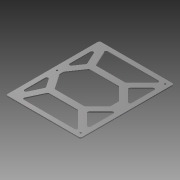
# Autodesk Inventor part: ZBedPlate
Saved by Autodesk Inventor 2015 SP1 (Build 190203100, 203)
## iProperties
Category: Sheet Metal
Created: 2015-01-11
Part Number: ZBedPlate
Material: Steel, Alloy
Document SubType Name: Modeling
Designer: Jack
Density: 7.73 g/cm^3
Appearance: Semi-Polished
Mass: 734.813 g
Surface Area: 727.52 cm^2
Volume: 95.0599 cm^3
Catalog Web Link: N/A
Author: Jack
Title: Bed Support Plate
Autodesk Inventor part; units mm, degrees
ref_plane "YZ Plane" through (0, 0, 0) normal (1, 0, 0) x (0, 1, 0)
ref_plane "XZ Plane" through (0, 0, 0) normal (0, 1, 0) x (-1, 0, 0)
ref_plane "XY Plane" through (0, 0, 0) normal (0, 0, 1) x (1, 0, 0)
sketch "Sketch1" plane through (0, 0, 0) normal (0, 0, 1) x (1, 0, 0)
  line L0 (0, 0) -> (236.5, 0)
  line L1 (236.5, 0) -> (236.5, 296)
  line L2 (236.5, 296) -> (0, 296)
  line L3 (0, 296) -> (0, 0)
  dimension "d0" = 236.5
  dimension "d1" = 296
  constraints: 8 end point, 2 parallel, 1 horizontal, 1 perpendicular
  measures "d0" distance of L0.start L0.end
  measures "d1" distance of L2.end L0.start
extrude "Extrusion1" add sketch "Sketch1" along normal blind 3
sketch "Sketch2" plane through (0, 0, 3) normal (0, 0, 1) x (1, 0, 0)
  line L0 (0, 0) -> (236.5, 0) projected
  line L1 (236.5, 0) -> (236.5, 296) projected
  line L2 (236.5, 296) -> (0, 296) projected
  line L3 (0, 296) -> (0, 0) projected
  line L4 (213.7907, 281) -> (33.7907, 281)
  line L5 (33.7907, 281) -> (60.8366, 223)
  line L6 (60.8366, 223) -> (155.5133, 223)
  line L7 (155.5133, 223) -> (213.7907, 281)
  line L8 (221.5, 260.4555) -> (173.8075, 212.9901)
  line L9 (173.8075, 212.9901) -> (221.5, 165.2976)
  line L10 (196.6646, 161.8487) -> (155.5133, 203)
  line L11 (221.5, 260.4555) -> (221.5, 165.2976)
  line L12 (155.5133, 203) -> (60.8366, 203)
  line L13 (60.8366, 203) -> (27.9297, 155)
  line L14 (15, 273.9728) -> (43.4367, 212.9901)
  line L15 (43.4367, 212.9901) -> (15, 171.5105)
  line L16 (15, 171.5105) -> (15, 273.9728)
  line L17 (27.9297, 141) -> (60.8366, 93)
  line L18 (60.8366, 93) -> (155.5133, 93)
  line L19 (155.5133, 93) -> (196.6646, 134.1513)
  line L20 (196.6646, 134.1513) -> (196.6646, 161.8487)
  line L21 (221.5, 130.7024) -> (173.8075, 83.0099)
  line L22 (173.8075, 83.0099) -> (221.5, 35.5445)
  line L23 (221.5, 35.5445) -> (221.5, 130.7024)
  line L24 (15, 124.4895) -> (43.4367, 83.0099)
  line L25 (43.4367, 83.0099) -> (15, 22.0272)
  line L26 (15, 22.0272) -> (15, 124.4895)
  line L27 (33.7907, 15) -> (213.7907, 15)
  line L28 (213.7907, 15) -> (155.5133, 73)
  line L29 (155.5133, 73) -> (60.8366, 73)
  line L30 (60.8366, 73) -> (33.7907, 15)
  line L31 (27.9297, 141) -> (27.9297, 155)
  dimension "d19" = 65
  dimension "d29" = 110
  dimension "d31" = 20
  dimension "d32" = 15
  dimension "d33" = 15
  dimension "d34" = 15
  dimension "d35" = 15
  dimension "d40" = 20
  dimension "d41" = 20
  dimension "d52" = 180
  dimension "d53" = 14
  dimension "d55" = 135
  dimension "d59" = 20
  dimension "d60" = 20
  dimension "d61" = 20
  dimension "d62" = 20
  dimension "d63" = 20
  constraints: 56 end point, 11 parallel, 9 vertical alignment, 8 equal length, 5 vertical, 4 horizontal, 2 horizontal alignment
  measures "d19" angle of L27 L30
  measures "d29" distance between parallel lines of L18 L12
  measures "d31" distance between parallel lines of L6 L12
  measures "d32" distance between parallel lines of L2 L4
  measures "d33" distance between parallel lines of L0 L27
  measures "d34" distance between parallel lines of L1 L11
  measures "d35" distance between parallel lines of L3 L16
  measures "d40" distance between parallel lines of L13 L15
  measures "d41" distance between parallel lines of L9 L10
  measures "d52" distance of L27.start L27.end
  measures "d53" distance of L17.start L13.end
  measures "d55" angle of L12 L10
  measures "d59" distance between parallel lines of L29 L18
  measures "d60" distance between parallel lines of L30 L25
  measures "d61" distance between parallel lines of L22 L28
  measures "d62" distance between parallel lines of L8 L7
  measures "d63" distance between parallel lines of L14 L5
extrude "Extrusion2" cut sketch "Sketch2" against normal up to next contours L7 L6 L5 L4 | L11 L9 L8 | L20 L19 L18 L17 L31 L13 L12 L10 | L14 L15 L16 | L23 L22 L21 | L24 L25 L26 | L30 L29 L28 L27
sketch "Sketch3" plane through (0, 0, 3) normal (0, 0, 1) x (1, 0, 0)
  line L0 (0, 0) -> (236.5, 0) projected
  line L1 (236.5, 0) -> (236.5, 296) projected
  line L2 (236.5, 296) -> (0, 296) projected
  line L3 (0, 296) -> (0, 0) projected
  circle A0 centre (222.5, 282) radius 2.75
  circle A1 centre (14, 148) radius 2.75
  circle A2 centre (222.5, 14) radius 2.75
  dimension "d44" = 5.5
  dimension "d45" = 14
  dimension "d46" = 14
  dimension "d47" = 14
  dimension "d56" = 148
  dimension "d57" = 14
  constraints: 3 centre point, 2 equal radius, 1 vertical alignment
  measures "d44" diameter of A0
  measures "d45" distance from line of L1 A0.centre
  measures "d46" distance from line of L2 A0.centre
  measures "d47" distance from line of L0 A2.centre
  measures "d56" distance from line of L2 A1.centre
  measures "d57" distance from line of L3 A1.centre
extrude "Extrusion3" cut sketch "Sketch3" against normal up to next contours A0 | A1 | A2
fillet "Fillet1" radius 4.7625 28 edges at (33.7907, 15, 1.5) (213.7907, 15, 1.5) (155.5133, 73, 1.5) (60.8366, 73, 1.5) (15, 22.0272, 1.5) (43.4367, 83.0099, 1.5) (15, 124.4895, 1.5) (43.4367, 212.9901, 1.5) (15, 171.5105, 1.5) (15, 273.9728, 1.5) (33.7907, 281, 1.5) (60.8366, 223, 1.5) (155.5133, 223, 1.5) (213.7907, 281, 1.5) (173.8075, 83.0099, 1.5) (221.5, 35.5445, 1.5) (221.5, 130.7024, 1.5) (221.5, 165.2976, 1.5) (173.8075, 212.9901, 1.5) (221.5, 260.4555, 1.5) (196.6646, 134.1513, 1.5) (196.6646, 161.8487, 1.5) (155.5133, 93, 1.5) (155.5133, 203, 1.5) (60.8366, 203, 1.5) (27.9297, 155, 1.5) (27.9297, 141, 1.5) (60.8366, 93, 1.5)
fillet "Fillet2" radius 5 4 edges at (236.5, 0, 1.5) (0, 0, 1.5) (0, 296, 1.5) (236.5, 296, 1.5)
body "Solid1"
